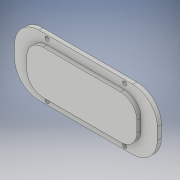
# Autodesk Inventor part: luz de freio
Saved by Autodesk Inventor 2019 (Build 230136000, 136)
## iProperties
Created: 2020-06-06
Part Number: luz de freio
Material: Genérico
Document SubType Name: Modeling
Designer: eliane
Density: 1 g/cm^3
Appearance: Padrão
Author: eliane
Autodesk Inventor part; units mm, degrees
ref_plane "YZ Plane" through (0, 0, 0) normal (1, 0, 0) x (0, 1, 0)
ref_plane "XZ Plane" through (0, 0, 0) normal (0, 1, 0) x (-1, 0, 0)
ref_plane "XY Plane" through (0, 0, 0) normal (0, 0, 1) x (1, 0, 0)
sketch "Esboço1" plane through (0, 0, 0) normal (0, 0, 1) x (1, 0, 0)
  line L0 (-29.6595, 42.7148) -> (-29.6595, -23.7852) construction
  line L1 (-29.6595, 42.7148) -> (65.3405, 42.7148) construction
  line L2 (65.3405, 42.7148) -> (65.3405, -23.7852) construction
  line L3 (65.3405, -23.7852) -> (-29.6595, -23.7852) construction
  circle A0 centre (65.3405, 42.7148) radius 2.5
  circle A1 centre (65.3405, -23.7852) radius 2.5
  circle A2 centre (-29.6595, 42.7148) radius 2.5
  circle A3 centre (-29.6595, -23.7852) radius 2.5
  line L4 (65.3405, 42.7148) -> (65.3405, 46.7148) construction
  line L5 (65.3405, 46.7148) -> (-29.6595, 46.7148) construction
  line L6 (-29.6595, 46.7148) -> (-29.6595, 42.7148) construction
  line L7 (65.3405, -23.7852) -> (65.3405, -27.7852) construction
  line L8 (65.3405, -27.7852) -> (-29.6595, -27.7852) construction
  line L9 (-29.6595, -27.7852) -> (-29.6595, -23.7852) construction
  line L10 (17.8405, 42.7148) -> (-37.1595, 42.7148) construction
  line L11 (17.8405, 42.7148) -> (72.8405, 42.7148) construction
  line L12 (17.8405, -23.7852) -> (-47.1595, -23.7852) construction
  line L13 (17.8405, -23.7852) -> (62.8405, -23.7852) construction
  line L14 (-29.6595, 46.7148) -> (-69.6595, 46.7148) construction
  line L15 (65.3405, -27.7852) -> (105.3405, -27.7852) construction
  line L16 (-39.6595, 46.7148) -> (75.3405, 46.7148)
  line L17 (105.3405, 16.7148) -> (105.3405, 2.2148)
  line L18 (75.3405, -27.7852) -> (-39.6595, -27.7852)
  line L19 (-69.6595, 2.2148) -> (-69.6595, 16.7148)
  arc A4 (-39.6595, 46.7148) -> (-69.6595, 16.7148) centre (-39.6595, 16.7148) ccw
  arc A5 (-69.6595, 2.2148) -> (-39.6595, -27.7852) centre (-39.6595, 2.2148) ccw
  arc A6 (105.3405, 16.7148) -> (75.3405, 46.7148) centre (75.3405, 16.7148) ccw
  arc A7 (75.3405, -27.7852) -> (105.3405, 2.2148) centre (75.3405, 2.2148) ccw
  dimension "d16" = 66.5
  dimension "d19" = 5
  dimension "d20" = 4
  dimension "d21" = 4
  dimension "d22" = 55
  dimension "d23" = 55
  dimension "d24" = 40
  dimension "d25" = 40
  dimension "d26" = 30
  dimension "d27" = 30
  constraints: 40 end point, 8 centre point, 8 point on circle, 8 tangent, 6 horizontal, 6 perpendicular, 6 point on line, 4 coincident, 4 vertical, 2 equal radius, 2 midpoint, 2 parallel
  measures "d16" distance of L0.start L0.end
  measures "d19" diameter of A0
  measures "d20" distance of L4.start L4.end
  measures "d21" distance of L7.start L7.end
  measures "d22" distance of L10.start L10.end
  measures "d23" distance of L10.start L11.end
  measures "d24" distance of L5.end L14.end
  measures "d25" distance of L7.end L15.end
  measures "d26" radius of A4
  measures "d27" radius of A5
extrude "Extrusão1" add sketch "Esboço1" along normal blind 5
sketch "Esboço2" plane through (0, 0, 5) normal (0, 0, 1) x (1, 0, 0)
  circle A0 centre (-29.6595, 42.7148) radius 2.5 construction
  line L0 (-29.6595, 40.2148) -> (-29.6595, 36.2148) construction
  circle A1 centre (65.3405, -23.7852) radius 2.5 construction
  line L1 (65.3405, -21.2852) -> (65.3405, -17.2852) construction
  line L2 (-29.6595, 36.2148) -> (-29.6595, 36.2148) construction
  line L3 (65.3405, -17.2852) -> (65.3405, -17.2852) construction
  line L4 (85.3405, 16.2148) -> (85.3405, 2.7148)
  line L5 (-49.6595, 2.7148) -> (-49.6595, 16.2148)
  arc A2 (-29.6595, 36.2148) -> (-49.6595, 16.2148) centre (-29.6595, 16.2148) ccw
  arc A3 (-49.6595, 2.7148) -> (-29.6595, -17.2852) centre (-29.6595, 2.7148) ccw
  arc A4 (85.3405, 16.2148) -> (65.3405, 36.2148) centre (65.3405, 16.2148) ccw
  arc A5 (65.3405, -17.2852) -> (85.3405, 2.7148) centre (65.3405, 2.7148) ccw
  line L6 (65.3405, 36.2148) -> (-29.6595, 36.2148)
  line L7 (-29.6595, -17.2852) -> (65.3405, -17.2852)
  point P0 (0, 0)
  dimension "d34" = 20
  constraints: 16 end point, 8 point on circle, 6 tangent, 4 centre point, 3 equal radius, 3 horizontal, 2 parallel, 2 vertical, 2 vertical alignment, 2 other
  measures "d34" radius of A2
extrude "Extrusão2" add sketch "Esboço2" along normal blind 5
sketch "Esboço3" plane through (0, 0, 0) normal (0, 0, -1) x (-1, 0, 0)
  circle A0 centre (-16.9737, 8.0827) radius 16.0131
  circle A1 centre (-16.9737, 8.0827) radius 11.1486
  point P0 (0, 0)
  constraints: 2 centre point, 1 coincident
extrude "Extrusão3" add sketch "Esboço3" along normal blind 10
sketch "Esboço4" plane through (16.9737, 8.0827, -10) normal (0, 0, -1) x (-1, 0, 0)
  circle A0 centre (-6.1571, -0.3724) radius 2
  circle A1 centre (6.017, -0.3724) radius 2
  point P0 (16.9737, -8.0827)
  dimension "d39" = 4
  constraints: 2 centre point
  measures "d39" diameter of A0
sketch "Esboço5" plane through (16.9737, 8.0827, -10) normal (0, 0, -1) x (-1, 0, 0)
  circle A0 centre (-6.1295, -0.4053) radius 1.2064
  circle A1 centre (5.9792, -0.4053) radius 1.3709
  point P0 (16.9737, -8.0827)
  constraints: 2 centre point
extrude "Extrusão4" add sketch "Esboço4" against normal blind 10
hole "Furo1" at (23.1031, 7.6774, -10) at (10.9944, 7.6774, -10) direction (0, 0, 1) diameter 3 depth 3 tip angle 118
